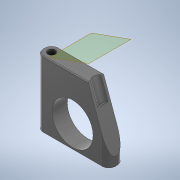
# Autodesk Inventor part: mid_mount_v3
Saved by Autodesk Inventor 2020 (Build 240168000, 168)
## iProperties
Created: 2024-02-03
Part Number: mid_mount_v3
Material: Пластик АБС
Document SubType Name: Modeling
Designer: 4s
Density: 1.06 g/cm^3
Appearance: Гладкая — черная
Author: 4s
Autodesk Inventor part; units mm, degrees
ref_plane "YZ Plane" through (0, 0, 0) normal (1, 0, 0) x (0, 1, 0)
ref_plane "XZ Plane" through (0, 0, 0) normal (0, 1, 0) x (-1, 0, 0)
ref_plane "XY Plane" through (0, 0, 0) normal (0, 0, 1) x (1, 0, 0)
sketch "Эскиз2" plane through (0, 0, 0) normal (0, 1, 0) x (-1, 0, 0)
  line L0 (19, -4) -> (-19, -4)
  line L1 (-19, -4) -> (-19, 4)
  line L2 (-19, 4) -> (19, 4)
  line L3 (19, 4) -> (19, -4)
  line L4 (19, -4) -> (-19, 4) construction
  line L5 (-19, -4) -> (19, 4) construction
  line L6 (19, 0) -> (-19, 0) construction
  circle A0 centre (-15, 0) radius 2
  line L7 (0, -4) -> (0, 4) construction
  circle A1 centre (15, 0) radius 2
  point P0 (0, 0)
  dimension "d1" = 30
  dimension "d2" = 4
  dimension "d3" = 38
  dimension "d4" = 8
  constraints: 16 end point, 6 midpoint, 2 centre point, 2 parallel, 1 horizontal, 1 perpendicular, 1 point on line, 1 symmetric about line, 1 other
  measures "d1" distance of A0.centre A1.centre
  measures "d2" diameter of A0
  measures "d3" distance of L1.end L2.end
  measures "d4" distance between parallel lines of L2 L0
extrude "Выдавливание1" add sketch "Эскиз2" along normal blind 35 contours L0 L1 L2 L3 | A0 | A1
fillet "Сопряжение1" radius 3.5 4 edges at (19, 17.5, 4) (19, 17.5, -4) (-19, 17.5, 4) (-19, 17.5, -4)
sketch "Эскиз3" plane through (-15.5, 0, 4) normal (0, 0, 1) x (1, 0, 0)
  line L0 (0, 0) -> (0, 35) construction
  line L1 (0, 0) -> (31, 0) construction
  line L2 (31, 35) -> (31, 0) construction
  line L3 (0, 35) -> (31, 35) construction
  line L4 (34.5, 35) -> (31, 35) construction
  line L5 (31, 35) -> (31, 0) construction
  line L6 (31, 0) -> (34.5, 0) construction
  line L7 (34.5, 0) -> (34.5, 35) construction
  line L8 (0, 35) -> (-3.5, 35) construction
  line L9 (-3.5, 35) -> (-3.5, 0) construction
  line L10 (-3.5, 0) -> (0, 0) construction
  line L11 (0, 0) -> (0, 35) construction
  line L12 (0, 0) -> (0, 35) construction
  line L13 (29, 35) -> (32, 35) construction
  line L14 (29, 0) -> (32, 0) construction
  line L15 (-1, 35) -> (2, 35) construction
  line L16 (-1, 0) -> (2, 0) construction
  line L17 (-1, 35) -> (2, 35) construction
  line L18 (-1, 0) -> (2, 0) construction
  line L19 (29, 35) -> (2, 0) construction
  line L20 (0, 35) -> (31, 35) construction
  line L21 (-3.5, 35) -> (0, 35) projected
  line L22 (0, 0) -> (31, 0) projected
  line L23 (0, 35) -> (31, 0) construction
  line L24 (15.5, 17.5) -> (15.5, 0) construction
  circle A0 centre (15.5, 12) radius 10.75
  dimension "d22" = 21.5
  dimension "d23" = 12
  constraints: 6 end point, 1 centre point, 1 midpoint, 1 point on line, 1 vertical, 1 other
  measures "d22" diameter of A0
  measures "d23" distance from line of L1 A0.centre
extrude "Выдавливание2" cut sketch "Эскиз3" against normal blind 35
sketch "Эскиз4" plane through (-15.5, 0, 4) normal (0, 0, 1) x (1, 0, 0)
  circle A0 centre (15.5, 12) radius 10.5 construction
  line L0 (0, 0) -> (0, 35) construction
  line L1 (0, 0) -> (31, 0) construction
  line L2 (31, 35) -> (31, 0) construction
  line L3 (0, 35) -> (31, 35) construction
  line L4 (0, 35) -> (-3.5, 35) construction
  line L5 (-3.5, 35) -> (-3.5, 0) construction
  line L6 (-3.5, 0) -> (0, 0) construction
  line L7 (0, 0) -> (0, 35) construction
  line L8 (34.5, 35) -> (31, 35) construction
  line L9 (31, 35) -> (31, 0) construction
  line L10 (31, 0) -> (34.5, 0) construction
  line L11 (34.5, 0) -> (34.5, 35) construction
  arc A1 (-1, 2.5793) -> (34.5, 12) centre (15.5, 12) ccw construction
  line L12 (-3.5, 0) -> (-3.5, 35) construction
  line L13 (34.5, 0) -> (34.5, 35) construction
  arc A2 (-3.5, 12) -> (-1, 2.5793) centre (15.5, 12) ccw construction
  line L14 (23.5012, 38.5457) -> (37.6912, 39.4976)
  line L15 (37.6912, 39.4976) -> (34.5, 5)
  circle A3 centre (15.5, 12) radius 15.5
  line L16 (34.5, 0) -> (31, 0) construction
  line L17 (34.5, 0) -> (34.5, 5) construction
  line L18 (34.5, 5) -> (23.6848, 35)
  line L19 (31, 35) -> (0, 35) construction
  line L20 (23.5012, 38.5457) -> (23.6848, 35)
  point P0 (15.5, 0)
  dimension "d18" = 5
  dimension "d24" = 31
  constraints: 10 end point, 4 point on circle, 4 point on line, 3 centre point, 2 tangent, 1 coincident
  measures "d18" distance of L10.end L15.end
  measures "d24" diameter of A3
extrude "Выдавливание3" cut sketch "Эскиз4" against normal blind 35 contours L14 L15 L18 L20
sketch "Эскиз5" plane through (0, 0, 0) normal (0, -1, 0) x (1, 0, 0)
  circle A0 centre (-15, 0) radius 2 projected
  circle A1 centre (15, 0) radius 2 projected
  point P0 (0, 0)
extrude "Выдавливание4" cut sketch "Эскиз5" against normal up to surface (35 mm away) contours A0
extrude "Выдавливание5" cut sketch "Эскиз5" against normal blind 10 contours A1
fillet "Сопряжение2" radius 0.5 14 edges at (-17.9749, 35, 2.9749) (-19, 35, 0) (-17.9749, 35, -2.9749) (-3.6576, 35, -4) (-3.6576, 35, 4) (8.1848, 35, 0) (17.9749, 0, 2.9749) (19, 0, 0) (17.9749, 0, -2.9749) (0, 0, -4) (-17.9749, 0, -2.9749) (-19, 0, 0) (-17.9749, 0, 2.9749) (0, 0, 4)
ref_plane "РабПлоскость1" through (-18.5, 35, 0) normal (0.3391, -0.9407, 0) x (0.9407, 0.3391, 0)
sketch "Эскиз6" plane through (-18.5, 35, 0) normal (0.3391, -0.9407, 0) x (0.9407, 0.3391, 0)
  ellipse E0 centre (23.0361, 0) end of major axis (23.0361, -2) minor radius 1.8815 construction
  ellipse E1 centre (19.6447, 0) end of major axis (19.6447, -2) minor radius 1.8815 construction
  line L0 (19.6447, 0) -> (23.0361, 0) construction
  circle A0 centre (27.2937, 0) radius 3.5
  point P0 (5.5337, 0)
  dimension "d26" = 7
  constraints: 2 end point, 1 centre point, 1 horizontal, 1 point on line, 2 other
  measures "d26" diameter of A0
extrude "Выдавливание6" cut sketch "Эскиз6" along normal blind 20
